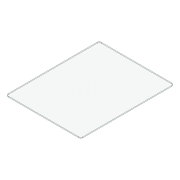
# Autodesk Inventor part: Puerta Lateral Izquierda
Saved by Autodesk Inventor 2020 (Build 240168000, 168)
## iProperties
Created: 2020-07-27
Part Number: Puerta Lateral Izquierda
Material: Genérico
Document SubType Name: Modeling
Designer: Pipi
Density: 1 g/cm^3
Appearance: Claro
Author: Pipi
Autodesk Inventor part; units mm, degrees
ref_plane "YZ Plane" through (0, 0, 0) normal (1, 0, 0) x (0, 1, 0)
ref_plane "XZ Plane" through (0, 0, 0) normal (0, 1, 0) x (-1, 0, 0)
ref_plane "XY Plane" through (0, 0, 0) normal (0, 0, 1) x (1, 0, 0)
sketch "Boceto1" plane through (0, 0, 0) normal (0, 1, 0) x (-1, 0, 0)
  line L0 (64.9389, -223.5898) -> (-165.0611, -223.5898)
  line L1 (-172.0611, -216.5898) -> (-172.0611, 73.4102)
  line L2 (-165.0611, 80.4102) -> (64.9389, 80.4102)
  line L3 (71.9389, 73.4102) -> (71.9389, -216.5898)
  arc A0 (-172.0611, -216.5898) -> (-165.0611, -223.5898) centre (-165.0611, -216.5898) ccw
  arc A1 (64.9389, -223.5898) -> (71.9389, -216.5898) centre (64.9389, -216.5898) ccw
  arc A2 (71.9389, 73.4102) -> (64.9389, 80.4102) centre (64.9389, 73.4102) ccw
  arc A3 (-165.0611, 80.4102) -> (-172.0611, 73.4102) centre (-165.0611, 73.4102) ccw
  point P0 (63.9389, -223.5898)
  point P1 (71.9389, -215.5898)
  point P2 (-172.0611, -215.5898)
  point P3 (-164.0611, -223.5898)
  point P4 (-172.0611, 72.4102)
  point P5 (-164.0611, 80.4102)
  point P6 (63.9389, 80.4102)
  point P7 (71.9389, 72.4102)
  dimension "d14" = 244
  dimension "d15" = 304
  dimension "d16" = 7
  constraints: 8 end point, 8 point on circle, 8 point on line, 8 tangent, 4 centre point, 3 equal radius, 2 parallel, 1 horizontal, 1 perpendicular
  measures "d14" distance between parallel lines of L1 L3
  measures "d15" distance between parallel lines of L0 L2
  measures "d16" radius of A0
extrude "Extrusión1" add sketch "Boceto1" along normal blind 3
